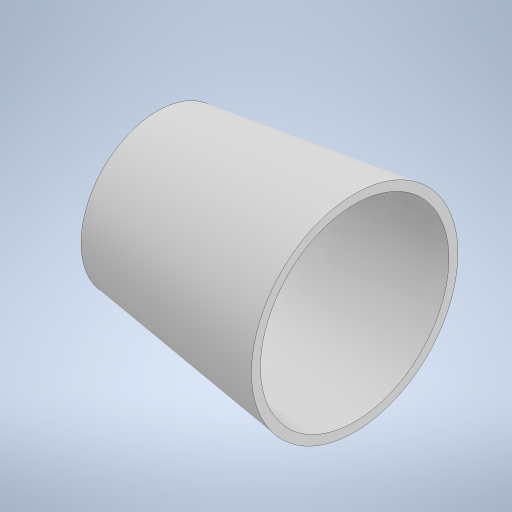
# Autodesk Inventor part: loft_example
Saved by Autodesk Inventor 2024 (Build 280153000, 153)
## iProperties
Created: 2024-03-07
Part Number: loft_example
Material: Generic
Document SubType Name: Modeling
Designer: Pintu
Density: 1 g/cm^3
Appearance: Default
Author: Pintu
Autodesk Inventor part; units mm, degrees
ref_plane "XZ Plane" through (0, 0, 0) normal (0, 1, 0) x (-1, 0, 0)
ref_plane "XY Plane" through (0, 0, 0) normal (0, 0, 1) x (1, 0, 0)
sketch "Sketch1" plane through (0, 0, 0) normal (1, 0, 0) x (0, 1, 0)
  circle A0 centre (0, 0) radius 37.5
  circle A1 centre (0, 0) radius 42.5
  dimension "d0" = 75
  dimension "d1" = 85
  constraints: 2 centre point, 2 coincident
  measures "d0" diameter of A0
  measures "d1" diameter of A1
ref_plane "Work Plane1" through (110, 0, 0) normal (1, 0, 0) x (0, 1, 0)
sketch "Sketch2" plane through (110, 0, 0) normal (1, 0, 0) x (0, 1, 0)
  circle A0 centre (0, 0) radius 52.5
  circle A1 centre (0, 0) radius 57.5
  dimension "d3" = 105
  dimension "d4" = 115
  constraints: 2 centre point, 2 coincident
  measures "d3" diameter of A0
  measures "d4" diameter of A1
loft "Loft1" add profiles "Sketch1", "Sketch2" contours A0 | A1 / A0 | A1
loft "Loft2" cut profiles "Sketch1", "Sketch2" contours A0 / A0
body "Solid1"
